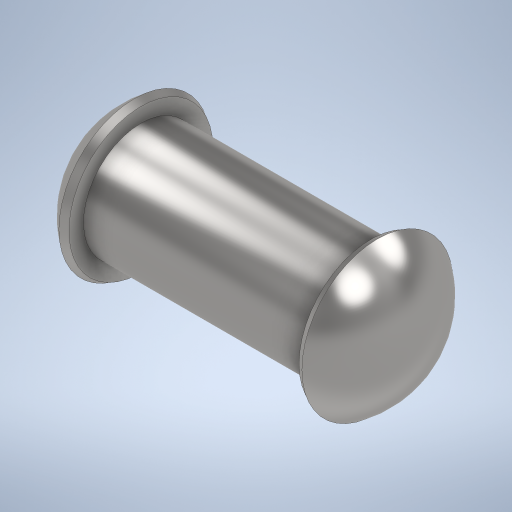
# Autodesk Inventor part: Claw Axis(1)
Saved by Autodesk Inventor 2024 (Build 280153000, 153)
## iProperties
Created: 2023-06-06
Part Number: Claw Axis(1)
Material: Stainless Steel
Document SubType Name: Modeling
Designer: vilas
Density: 8 g/cm^3
Appearance: Semi-Polished
Author: vilas
Autodesk Inventor part; units mm, degrees
ref_plane "YZ Plane" through (0, 0, 0) normal (1, 0, 0) x (0, 1, 0)
ref_plane "XZ Plane" through (0, 0, 0) normal (0, 1, 0) x (-1, 0, 0)
ref_plane "XY Plane" through (0, 0, 0) normal (0, 0, 1) x (1, 0, 0)
sketch "Sketch1" plane through (0, 0, 0) normal (0, 0, 1) x (1, 0, 0)
  line L0 (0, 0) -> (15, 0)
  line L1 (15, 0) -> (15, 3.75)
  line L2 (15, 3.75) -> (0, 3.75)
  line L3 (0, 3.75) -> (0, 0)
  line L4 (0, 3.75) -> (0, 5.1962)
  line L5 (15, 3.75) -> (15, 5.1962)
  arc A0 (18, 0) -> (15, 5.1962) centre (12, 0) ccw
  arc A1 (0, 5.1962) -> (-3, 0) centre (3, 0) ccw
  line L6 (0, 0) -> (-3, 0)
  line L7 (15, 0) -> (18, 0)
  dimension "d0" = 15
  dimension "d1" = 3.75
  dimension "d2" = 6
  dimension "d3" = 6
  dimension "d4" = 3
  dimension "d5" = 3
  constraints: 16 end point, 4 point on circle, 3 horizontal, 2 centre point, 2 parallel, 2 point on line, 2 vertical, 1 perpendicular
  measures "d0" distance of L2.end L1.end
  measures "d1" distance of L1.end L0.end
  measures "d2" radius of A0
  measures "d3" radius of A1
  measures "d4" distance of A0.centre L0.end
  measures "d5" distance of A1.centre L0.start
revolve "Revolution1" add sketch "Sketch1" angle 360 about axis through (0, 0, 0) along (1, 0, 0)
chamfer "Chamfer1" distance 0.5 angle 45 2 edges at (0, -5.1962, 0) (15, -5.1962, 0)
body "Solid1"
